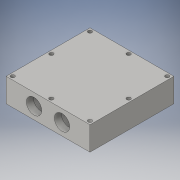
# Autodesk Inventor part: water_block_top
Saved by Autodesk Inventor 2016 (Build 200138000, 138)
## iProperties
Created: 2016-02-26
Part Number: water_block_top
Material: Generic
Document SubType Name: Modeling
Designer: USKHNGO
Density: 1 g/cm^3
Appearance: Default
Author: USKHNGO
Autodesk Inventor part; units mm, degrees
ref_plane "YZ Plane" through (0, 0, 0) normal (1, 0, 0) x (0, 1, 0)
ref_plane "XZ Plane" through (0, 0, 0) normal (0, 1, 0) x (-1, 0, 0)
ref_plane "XY Plane" through (0, 0, 0) normal (0, 0, 1) x (1, 0, 0)
sketch "Sketch1" plane through (0, 0, 0) normal (0, 1, 0) x (-1, 0, 0)
  line L0 (0, 0) -> (-76.2, 0)
  line L1 (-76.2, 0) -> (-76.2, -76.2)
  line L2 (-76.2, -76.2) -> (0, -76.2)
  line L3 (0, -76.2) -> (0, 0)
  dimension "d0" = 76.2
  dimension "d1" = 76.2
  constraints: 8 end point, 2 parallel, 1 horizontal, 1 perpendicular
  measures "d0" distance of L2.end L1.end
  measures "d1" distance of L1.end L0.end
extrude "Extrusion1" add sketch "Sketch1" along normal blind 21.59
sketch "Sketch2" plane through (0, 21.59, 0) normal (0, 1, 0) x (1, 0, 0)
  line L0 (76.2, 76.2) -> (0, 76.2) projected
  line L1 (38.1, 76.2) -> (38.1, 73.1774)
  line L2 (0, 76.2) -> (0, 0) projected
  line L3 (0, 38.1) -> (3.0226, 38.1)
  line L4 (0, 0) -> (76.2, 0) projected
  line L5 (38.1, 0) -> (38.1, 3.0226)
  line L6 (76.2, 0) -> (76.2, 76.2) projected
  line L7 (76.2, 38.1) -> (73.1774, 38.1)
  circle A0 centre (3.0226, 73.1774) radius 1.7526
  circle A1 centre (73.1774, 3.0226) radius 1.7526
  circle A2 centre (73.1774, 73.1774) radius 1.7526
  circle A3 centre (38.1, 3.0226) radius 1.7526
  circle A4 centre (3.0226, 38.1) radius 1.7526
  circle A5 centre (38.1, 73.1774) radius 1.7526
  circle A6 centre (3.0226, 3.0226) radius 1.7526
  circle A7 centre (73.1774, 38.1) radius 1.7526
  dimension "d5" = 3.0226
  dimension "d6" = 3.0226
  dimension "d7" = 3.0226
  dimension "d8" = 3.0226
  dimension "d9" = 3.5052
  dimension "d10" = 3.5052
  dimension "d11" = 3.5052
  dimension "d12" = 3.5052
  dimension "d13" = 3.5052
  dimension "d14" = 3.5052
  dimension "d15" = 3.5052
  dimension "d16" = 3.5052
  constraints: 8 centre point, 8 end point, 4 midpoint, 2 horizontal, 2 vertical
  measures "d5" distance of L1.start L1.end
  measures "d6" distance of L3.start L3.end
  measures "d7" distance of L5.start L5.end
  measures "d8" distance of L7.start L7.end
  measures "d9" diameter of A0
  measures "d10" diameter of A1
  measures "d11" diameter of A2
  measures "d12" diameter of A3
  measures "d13" diameter of A4
  measures "d14" diameter of A5
  measures "d15" diameter of A6
  measures "d16" diameter of A7
extrude "Extrusion2" cut sketch "Sketch2" against normal blind 11.43 contours A5 | A4 | A3 | A7 | A0 | A1 | A2 | A6
sketch "Sketch3" plane through (0, 0, 0) normal (0, 0, 1) x (1, 0, 0)
  line L0 (0, 0) -> (0, 21.59) projected
  circle A0 centre (25.4, 10.795) radius 6.985
  circle A1 centre (50.8, 10.795) radius 6.985
  dimension "d21" = 13.97
  dimension "d22" = 13.97
  constraints: 2 centre point
  measures "d21" diameter of A0
  measures "d22" diameter of A1
extrude "Extrusion3" cut sketch "Sketch3" against normal blind 6.35
body "Solid1"
